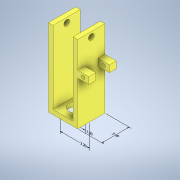
# Autodesk Inventor part: forkV02
Saved by Autodesk Inventor 2021.1 (Build 251245000, 245)
## iProperties
Created: 2020-07-21
Part Number: forkV02
Material: PC/ABS Plastic
Document SubType Name: Modeling
Designer: robst
Density: 0.357273 g/cm^3
Appearance: Smooth - Yellow
Mass: 137.886 g
Surface Area: 962.27 cm^2
Volume: 385.941 cm^3
Author: robst
Autodesk Inventor part; units mm, degrees
ref_plane "YZ Plane" through (0, 0, 0) normal (1, 0, 0) x (0, 1, 0)
ref_plane "XZ Plane" through (0, 0, 0) normal (0, 1, 0) x (-1, 0, 0)
ref_plane "XY Plane" through (0, 0, 0) normal (0, 0, 1) x (1, 0, 0)
sketch "Sketch1" plane through (0, 0, 0) normal (0, 0, 1) x (1, 0, 0)
  line L0 (0, 0) -> (27.94, 0)
  line L1 (27.94, 0) -> (27.94, 203.2)
  line L2 (0, 0) -> (-27.94, 0)
  line L3 (-27.94, 0) -> (-27.94, 203.2)
  line L4 (-27.94, 203.2) -> (-40.64, 203.2)
  line L5 (-40.64, 203.2) -> (-40.64, -12.7)
  line L6 (-40.64, -12.7) -> (40.64, -12.7)
  line L7 (40.64, -12.7) -> (40.64, 203.2)
  line L8 (40.64, 203.2) -> (27.94, 203.2)
  dimension "d0" = 203.2
  dimension "d1" = 27.94
  dimension "x2" = 12.7
  dimension "d3" = 12.7
  dimension "d4" = 12.7
  constraints: 18 end point, 5 perpendicular, 3 horizontal, 2 equal length, 1 point on line, 1 vertical
  measures "d0" distance of L0.end L1.end
  measures "d1" distance from line of L1 L0.start
  measures "x2" distance between parallel lines of L5 L3
  measures "d3" distance between parallel lines of L2 L6
  measures "d4" distance of L7.end L1.end
extrude "Extrusion1" add sketch "Sketch1" against normal mid plane 76.2
sketch "Sketch2" plane through (40.64, -12.7, -38.1) normal (1, 0, 0) x (0, 0, -1)
  circle A0 centre (-38.1, 203.2) radius 7.9375
  point P0 (-38.1, 12.7)
  dimension "d7" = 15.875
  dimension "d8" = 190.5
  constraints: 1 centre point
  measures "d7" diameter of A0
  measures "d8" distance of A0.centre point (-38.1, 12.7)
extrude "Extrusion2" cut sketch "Sketch2" against normal through all
sketch "Sketch3" plane through (0, 0, 38.1) normal (0, 0, 1) x (1, 0, 0)
  line L0 (40.64, 203.2) -> (40.64, -12.7) projected
  line L1 (40.64, 129.286) -> (72.39, 129.286)
  line L2 (72.39, 129.286) -> (72.39, 110.236)
  line L3 (72.39, 110.236) -> (40.64, 110.236)
  line L4 (40.64, 110.236) -> (40.64, 129.286)
  line L5 (40.64, 119.761) -> (72.39, 119.761) construction
  line L6 (-40.64, -12.7) -> (40.64, -12.7) construction
  circle A0 centre (56.3118, 119.761) radius 4.7625
  point P0 (0, 0)
  point P1 (40.64, 110.236)
  dimension "d20" = 31.75
  dimension "d21" = 19.05
  dimension "d22" = 132.461
  dimension "d23" = 9.525
  dimension "d24" = 15.6718
  constraints: 10 end point, 2 midpoint, 2 parallel, 2 point on line, 1 centre point, 1 horizontal, 1 perpendicular
  measures "d20" distance of L2.end L3.end
  measures "d21" distance of L1.end L2.end
  measures "d22" distance between parallel lines of L5 L6
  measures "d23" diameter of A0
  measures "d24" distance from line of A0.centre L0
extrude "Extrusion3" add sketch "Sketch3" against normal blind 19.05
mirror "Mirror1" about plane through (0, 0, 0) normal (0, 0, 1) of "Extrusion3"
sketch "Sketch4" plane through (-40.64, -12.7, -38.1) normal (0, -1, 0) x (1, 0, 0)
  circle A0 centre (40.64, 38.1) radius 20.6375
  dimension "d27" = 41.275
  constraints: 1 centre point, 1 coincident
  measures "d27" diameter of A0
extrude "Extrusion4" cut sketch "Sketch4" against normal through all
equation "\"d0\" = overallHeight"
equation "\"x2\" = wallThickness"
equation "\"d3\" = wallThickness"
equation "\"d4\" = wallThickness"
equation "\"d5\" = overallWidth"
equation "\"d7\" = postHoleDiameter"
equation "\"d8\" = postHoleFromTop"
equation "\"postHoleDiameter\" = 15.875"
equation "\"overallHeight\" = 203.2"
equation "\"wallThickness\" = 12.7"
equation "\"overallWidth\" = 76.2"
equation "\"postHoleFromTop\" = 190.5"
body "Solid1"
